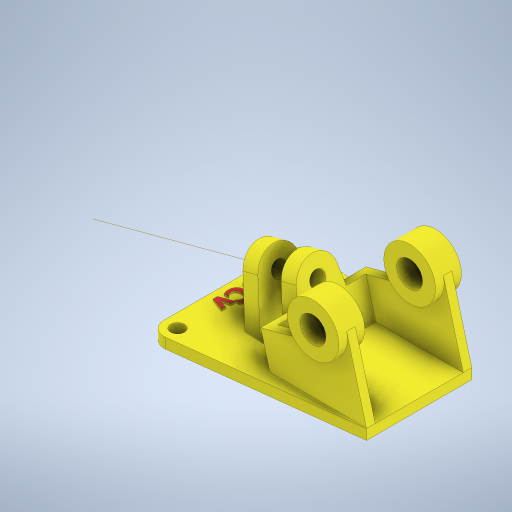
# Autodesk Inventor part: Reper
Saved by Autodesk Inventor 2024 (Build 280153000, 153)
## iProperties
Created: 2024-03-05
Part Number: Reper
Material: Steel, Carbon
Document SubType Name: Modeling
Designer: alexa
Density: 7.85 g/cm^3
Appearance: Canary
Author: alexa
Autodesk Inventor part; units mm, degrees
ref_plane "YZ Plane" through (0, 0, 0) normal (1, 0, 0) x (0, 1, 0)
ref_plane "XZ Plane" through (0, 0, 0) normal (0, 1, 0) x (-1, 0, 0)
ref_plane "XY Plane" through (0, 0, 0) normal (0, 0, 1) x (1, 0, 0)
sketch "Sketch1" plane through (0, 0, 0) normal (0, 0, 1) x (1, 0, 0)
  line L0 (-24.2255, 0) -> (145.3528, 0) projected
  line L1 (-24.6963, -6.6174) -> (148.1779, 39.7041) projected
  line L2 (78.9979, 33.5907) -> (87.6912, 35.9201)
  line L3 (87.6912, 35.9201) -> (96.4453, 3.2495)
  line L4 (96.4453, 3.2495) -> (109.9682, 6.873)
  line L5 (109.9682, 6.873) -> (101.2142, 39.5436)
  line L6 (101.2142, 39.5436) -> (109.9075, 41.8729)
  line L7 (109.9075, 41.8729) -> (121.1273, 0)
  line L8 (121.1273, 0) -> (87.9985, 0)
  line L9 (87.9985, 0) -> (78.9979, 33.5907)
  point P0 (0, 0)
  point P1 (121.1273, 0)
  dimension "d0" = 9
  dimension "d1" = 9
  dimension "d2" = 12
  dimension "d3" = 117
  dimension "d4" = 14
  dimension "d5" = 35
  constraints: 16 end point, 4 perpendicular, 2 parallel, 2 point on line, 1 collinear, 1 horizontal
  measures "d0" distance of L2.start L2.end
  measures "d1" distance of L5.end L6.end
  measures "d2" distance from line of L6.end L1
  measures "d3" distance from line of L7 point (0, 0)
  measures "d4" distance between parallel lines of L5 L3
  measures "d5" distance of L2.start L3.end
extrude "Extrusion1" add sketch "Sketch1" along normal mid plane 50 contours L9 L1 L3 L4 L5 L7 L0 | L9 L2 L3 L1 | L1 L5 L6 L7
sketch "Sketch2" plane through (87.9985, 0, -25) normal (-0.9659258, -0.258819, 0) x (0, 0, 1)
  line L0 (25, 56.0118) -> (25, -35.6665) projected
  line L1 (0, 34.7757) -> (50, 34.7757) projected
  line L2 (0, -8.5744) -> (50, -8.5744) projected
  line L3 (4.7024, -15) -> (13.2622, 25.2706)
  arc A0 (25, 34.7757) -> (13.2622, 25.2706) centre (25, 22.7757) ccw
  line L4 (4.7024, -15) -> (45.2976, -15)
  line L5 (45.2976, -15) -> (36.7378, 25.2706)
  arc A1 (36.7378, 25.2706) -> (25, 34.7757) centre (25, 22.7757) ccw
  line L6 (0, 0) -> (50, 0) projected
  point P0 (25, -15)
  point P1 (25, 34.7757)
  dimension "d8" = 12
  dimension "d9" = 78
  dimension "d10" = 78
  dimension "d11" = 15
  constraints: 6 end point, 4 point on circle, 4 tangent, 3 midpoint, 2 centre point, 2 coincident, 1 horizontal
  measures "d8" radius of A0
  measures "d11" distance between parallel lines of L6 L4
extrude "Extrusion2" cut sketch "Sketch2" against normal blind 50 keep common part
sketch "Sketch5" plane through (0, 0, 0) normal (0, 0, 1) x (1, 0, 0)
  line L0 (-24.2255, 0) -> (145.3528, 0) projected
  line L1 (-24.6963, -6.6174) -> (148.1779, 39.7041) projected
  line L2 (108.5423, 19.4508) -> (133.7742, 26.2117)
  line L3 (133.7742, 26.2117) -> (131.3659, 35.1994)
  line L4 (131.3659, 35.1994) -> (160.3437, 42.964)
  line L5 (160.3437, 42.964) -> (171.8558, 0)
  line L6 (171.8558, 0) -> (115.9509, 0)
  line L7 (115.9509, 0) -> (110.5919, 20)
  line L8 (112.3676, 32.6918) -> (121.1273, 0) projected
  line L9 (109.9075, 41.8729) -> (112.3676, 32.6918) projected
  point P0 (0, 0)
  point P1 (132.57, 30.7055)
  point P2 (171.8558, 0)
  point P3 (115.9509, 0)
  dimension "d23" = 5
  dimension "d24" = 20
  dimension "d25" = 30
  dimension "d26" = 49
  constraints: 12 end point, 5 perpendicular, 2 collinear, 1 horizontal, 1 midpoint, 1 point on line
  measures "d23" distance between parallel lines of L8 L7
  measures "d24" vertical distance of L6.end L7.end
  measures "d25" distance from line of L5 point (132.57, 30.706)
  measures "d26" distance between parallel lines of L5 L9
extrude "Extrusion5" add sketch "Sketch5" along normal mid plane 61 contours L7 L2 L8 L0 | L8 L2 L3 L1 L4 L5 L6 L0
sketch "Sketch6" plane through (131.3659, 35.1994, 30.5) normal (-0.258819, 0.9659258, 0) x (0.9659258, 0.258819, 0)
  line L0 (-19, 56) -> (35, 56)
  line L1 (35, 56) -> (35, 5)
  line L2 (35, 5) -> (-19, 5)
  line L3 (-19, 5) -> (-19, 56)
  line L4 (-24, 61) -> (0, 61) projected
  line L5 (-24, 16.2541) -> (-24, 0) projected
  line L6 (30, 0) -> (0, 0) projected
  line L7 (30, 61) -> (30, 0) projected
  point P0 (-136, 30.5)
  point P1 (30, 5)
  point P2 (30, 56)
  dimension "d29" = 5
  dimension "d30" = 5
  dimension "d31" = 5
  dimension "d32" = 5
  constraints: 8 end point, 2 parallel, 1 horizontal, 1 perpendicular
  measures "d29" distance between parallel lines of L4 L0
  measures "d30" distance between parallel lines of L3 L5
  measures "d31" distance between parallel lines of L6 L2
  measures "d32" distance between parallel lines of L7 L1
extrude "Extrusion6" cut sketch "Sketch6" against normal blind 61 contours L0 L7 L2 L3
sketch "Sketch7" plane through (0, 0, 0) normal (0, 0, 1) x (1, 0, 0)
  circle A0 centre (145.8548, 39.0817) radius 15
  line L0 (131.3659, 35.1994) -> (160.3437, 42.964) projected
  point P0 (0, 0)
  dimension "d35" = 30
  constraints: 1 centre point, 1 coincident, 1 midpoint
  measures "d35" diameter of A0
extrude "Extrusion7" add sketch "Sketch7" along normal mid plane 71
sketch "Sketch8" plane through (0, 0, 0) normal (0, 0, 1) x (1, 0, 0)
  circle A0 centre (145.8548, 39.0817) radius 19.5
  circle A1 centre (145.8548, 39.0817) radius 15 projected
  point P0 (0, 0)
  dimension "d38" = 39
  constraints: 1 centre point, 1 concentric
  measures "d38" diameter of A0
extrude "Extrusion8" cut sketch "Sketch8" along normal mid plane 41 contours A0 | A1
sketch "Sketch9" plane through (0, 0, 0) normal (0, 1, 0) x (-1, 0, 0)
  line L0 (-206.227, 0) -> (34.3712, 0) projected
  line L1 (-58.8558, -35) -> (-58.8558, 35)
  line L2 (-67.8058, 42.9434) -> (-171.8558, 30.5)
  line L3 (-171.8558, 30.5) -> (-171.8558, -30.5)
  line L4 (-171.8558, -30.5) -> (-67.8058, -42.9434)
  arc A0 (-67.8058, -42.9434) -> (-58.8558, -35) centre (-66.8558, -35) ccw
  arc A1 (-58.8558, 35) -> (-67.8058, 42.9434) centre (-66.8558, 35) ccw
  point P0 (0, 0)
  dimension "d41" = 8
  dimension "d42" = 113
  dimension "d43" = 70
  dimension "d44" = 35
  constraints: 8 end point, 4 point on circle, 4 tangent, 2 centre point, 2 coincident, 1 equal radius, 1 vertical
  measures "d41" radius of A0
  measures "d42" distance between parallel lines of L3 L1
  measures "d43" distance of A1.centre A0.centre
  measures "d44" distance from line of L0 A0.centre
extrude "Extrusion9" add sketch "Sketch9" against normal blind 6
sketch "Sketch10" plane through (145.8548, 39.0817, 35.5) normal (0, 0, 1) x (1, 0, 0)
  circle A0 centre (0, 0) radius 15 projected
  point P0 (-145.8548, -39.0817)
  constraints: 1 coincident
hole "Hole1" at (145.8548, 39.0817, 35.5) direction (0, 0, -1) diameter 15 end through all
sketch "Sketch11" plane through (82.1037, 21.9996, 0) normal (-0.9659258, -0.258819, 0) x (0, 0, 1)
  arc A0 (11.7378, 2.4949) -> (-11.7378, 2.4949) centre (0, 0) ccw projected
  constraints: 1 coincident
hole "Hole2" at (82.1037, 21.9996, 0) at (82.1037, 21.9996, 0) direction (0.9659258, 0.258819, 0) diameter 9 end through all
sketch "Sketch12" plane through (0, 0, 0) normal (0, 1, 0) x (1, 0, 0)
  arc A0 (67.8058, 42.9434) -> (58.8558, 35) centre (66.8558, 35) ccw projected
  point P0 (0, 0)
  constraints: 1 coincident
hole "Hole3" at (66.8558, 0, -35) direction (0, -1, 0) diameter 8 end through all
sketch "Sketch13" plane through (0, 0, 0) normal (0, 1, 0) x (1, 0, 0)
  arc A0 (58.8558, -35) -> (67.8058, -42.9434) centre (66.8558, -35) ccw projected
  point P0 (0, 0)
  constraints: 1 coincident
hole "Hole4" at (66.8558, 0, 35) direction (0, -1, 0) diameter 8 end through all
sketch "Sketch14" plane through (0, 0, 0) normal (0, 1, 0) x (1, 0, 0)
  line L0 (73.8558, 14.5) -> (73.8558, -14.5) construction
  line L1 (73.8558, -14.5) -> (62.8558, -14.5) construction
  line L2 (62.8558, -14.5) -> (62.8558, 14.5) construction
  line L3 (62.8558, 14.5) -> (73.8558, 14.5) construction
  line L4 (58.8558, 35) -> (58.8558, -35) projected
  spline S0 degree 2 poles (63.1533, 8.5697) (63.1533, 10.5875) (65.0981, 12.7593) (66.9782, 12.7593) knots 0 0 0 1 2 2 2
  line L5 (66.9782, 12.7593) -> (73.364, 12.7593)
  line L6 (73.364, 12.7593) -> (73.364, 10.2472)
  line L7 (73.364, 10.2472) -> (67.1241, 10.2472)
  spline S1 degree 2 poles (67.1241, 10.2472) (66.0787, 10.2472) (65.0576, 9.4611) (65.0576, 8.5697) knots 0 0 0 1 2 2 2
  spline S2 degree 2 poles (65.0576, 8.5697) (65.0576, 7.7026) (66.0382, 6.8922) (67.1241, 6.8922) knots 0 0 0 1 2 2 2
  line L8 (67.1241, 6.8922) -> (73.364, 6.8922)
  line L9 (73.364, 6.8922) -> (73.364, 4.3801)
  line L10 (73.364, 4.3801) -> (66.9863, 4.3801)
  spline S3 degree 2 poles (66.9863, 4.3801) (65.1387, 4.3801) (63.1533, 6.4951) (63.1533, 8.5697) knots 0 0 0 1 2 2 2
  spline S4 degree 2 poles (63.1695, -1.8598) (63.1695, 0.393) (65.8923, 3.0348) (68.3558, 3.0348) knots 0 0 0 1 2 2 2
  spline S5 degree 2 poles (68.3558, 3.0348) (70.7302, 3.0348) (73.5584, 0.3849) (73.5584, -1.8679) knots 0 0 0 1 2 2 2
  spline S6 degree 2 poles (73.5584, -1.8679) (73.5584, -2.4595) (73.4207, -3.4157) (73.3072, -3.8533) knots 0 0 0 1 2 2 2
  spline S7 degree 2 poles (73.3072, -3.8533) (73.2019, -4.1937) (72.8534, -4.9959) (72.7238, -5.2472) knots 0 0 0 1 2 2 2
  line L11 (72.7238, -5.2472) -> (70.3413, -5.2472)
  line L12 (70.3413, -5.2472) -> (70.3413, -4.9959)
  spline S8 degree 2 poles (70.3413, -4.9959) (70.5033, -4.8096) (70.9571, -4.2585) (71.1678, -3.91) knots 0 0 0 1 2 2 2
  spline S9 degree 2 poles (71.1678, -3.91) (71.3866, -3.5616) (71.6865, -2.7269) (71.6865, -2.265) knots 0 0 0 1 2 2 2
  spline S10 degree 2 poles (71.6865, -2.265) (71.6865, -1.722) (71.3461, -0.8225) (70.9166, -0.4092) knots 0 0 0 1 2 2 2
  spline S11 degree 2 poles (70.9166, -0.4092) (70.5357, -0.0365) (69.231, 0.4417) (68.3477, 0.4417) knots 0 0 0 1 2 2 2
  spline S12 degree 2 poles (68.3477, 0.4417) (67.4158, 0.4417) (66.1435, -0.0527) (65.7545, -0.4579) knots 0 0 0 1 2 2 2
  spline S13 degree 2 poles (65.7545, -0.4579) (65.3737, -0.8468) (65.0414, -1.8031) (65.0414, -2.2812) knots 0 0 0 1 2 2 2
  spline S14 degree 2 poles (65.0414, -2.2812) (65.0414, -2.7755) (65.3737, -3.675) (65.5763, -3.983) knots 0 0 0 1 2 2 2
  spline S15 degree 2 poles (65.5763, -3.983) (65.7789, -4.3233) (66.2084, -4.8339) (66.3785, -5.0203) knots 0 0 0 1 2 2 2
  line L13 (66.3785, -5.0203) -> (66.3785, -5.2472)
  line L14 (66.3785, -5.2472) -> (64.0285, -5.2472)
  spline S16 degree 2 poles (64.0285, -5.2472) (63.8988, -4.9716) (63.5746, -4.2504) (63.4612, -3.8614) knots 0 0 0 1 2 2 2
  spline S17 degree 2 poles (63.4612, -3.8614) (63.3153, -3.3914) (63.1695, -2.5729) (63.1695, -1.8598) knots 0 0 0 1 2 2 2
  line L15 (70.9085, -13.6507) -> (63.364, -10.9441)
  line L16 (63.364, -10.9441) -> (63.364, -8.3752)
  line L17 (63.364, -8.3752) -> (70.9085, -5.6929)
  line L18 (70.9085, -5.6929) -> (70.9085, -8.1645)
  line L19 (70.9085, -8.1645) -> (65.9247, -9.7042)
  line L20 (65.9247, -9.7042) -> (70.9085, -11.2277)
  line L21 (70.9085, -11.2277) -> (70.9085, -13.6507)
  point P0 (0, 0)
  point P1 (62.8558, 0)
  point P2 (58.8558, 0)
  dimension "d75" = 15
  dimension "d76" = 29
  dimension "d77" = 11
  constraints: 2 midpoint, 1 horizontal alignment, 1 parallel, 2 other
  measures "d75" distance from line of L4 L0.start
  measures "d76" distance between parallel lines of L1 L3
  measures "d77" distance between parallel lines of L2 L0
emboss "Emboss1" sketch "Sketch14" operation add depth 1 direction (0, -1, 0)
equation "\"d35\" = d25"
equation "\"d38\" = 1.3 * d25"
equation "\"d44\" = 0.5 * d43"
body "Solid1"
